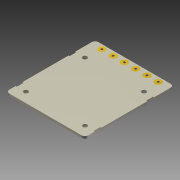
# Autodesk Inventor part: SLIPRING_SRG-1-6G_
Saved by Autodesk Inventor 2011 (Build 150239000, 239)
## iProperties
Created: 2012-05-23
Part Number: SLIPRING_SRG-1-6G_
Document SubType Name: Modeling
Designer: arihon
Density: 1 g/cm^3
Author: arihon
Autodesk Inventor part; units mm, degrees
ref_plane "YZ Plane" through (0, 0, 0) normal (1, 0, 0) x (0, 1, 0)
ref_plane "XZ Plane" through (0, 0, 0) normal (0, 1, 0) x (-1, 0, 0)
ref_plane "XY Plane" through (0, 0, 0) normal (0, 0, 1) x (1, 0, 0)
sketch "スケッチ1" plane through (0, 0, 0) normal (0, 0, 1) x (1, 0, 0)
  circle A0 centre (13.0815, -13.0815) radius 1
  circle A1 centre (-13.0815, 13.0815) radius 1
  circle A2 centre (13.0815, 13.0815) radius 1
  line L0 (-17.5, -17.5) -> (17.5, -17.5)
  line L1 (17.5, -17.5) -> (17.5, -13.2)
  line L2 (17.5, 22) -> (-17.5, 22)
  line L3 (-17.5, 22) -> (-17.5, 13.2505)
  line L4 (-17.0382, 13.2505) -> (-17.5, 13.2505)
  line L5 (-17.5, 13.2505) -> (-17.5, 13.2)
  line L6 (-17.5, 10.2) -> (-17.0382, 10.2)
  line L7 (-17.0382, 10.2) -> (-17.0382, 13.2505)
  line L8 (-17, -10.2) -> (-17.5, -10.2)
  line L9 (-17.5, -10.2) -> (-17.5, -13.2)
  line L10 (-17.5, -13.2) -> (-17, -13.2)
  line L11 (-17, -13.2) -> (-17, -10.2)
  line L12 (17.5, -10.2) -> (17, -10.2)
  line L13 (17, -10.2) -> (17, -13.2)
  line L14 (17, -13.2) -> (17.5, -13.2)
  line L15 (17.5, -13.2) -> (17.5, -10.2)
  line L16 (17.5, 13.2) -> (17, 13.2)
  line L17 (17, 13.2) -> (17, 10.2)
  line L18 (17, 10.2) -> (17.5, 10.2)
  line L19 (17.5, 10.2) -> (17.5, 13.2)
  line L20 (17, 13.2) -> (17.5, 13.2)
  line L21 (17.5, 13.2) -> (17.5, 22)
  line L22 (17.5, 10.2) -> (17.5, 13.2)
  line L23 (17.5, -10.2) -> (17.5, 10.2)
  line L24 (17.5, -13.2) -> (17.5, -10.2)
  line L25 (-17.5, -13.2) -> (-17.5, -17.5)
  line L26 (-17.5, -10.2) -> (-17.5, -13.2)
  line L27 (-17.5, 13.2505) -> (-17.5, 13.2)
  line L28 (-17.5, 13.2) -> (-17.5, 10.2)
  line L29 (-17.5, 10.2) -> (-17.5, -10.2)
  line L30 (-17.5, 13.2) -> (-17.5, 10.2)
  circle A3 centre (-13.0815, 13.0815) radius 1
  circle A4 centre (13.0815, 13.0815) radius 1
  circle A5 centre (-13.0815, -13.0815) radius 1
  circle A6 centre (13.0815, -13.0815) radius 1
  circle A7 centre (-13.0815, -13.0815) radius 1
  point P0 (0, 0)
  point P1 (0, 0)
  dimension "d0" = 39.5
  dimension "d1" = 2
  constraints: 63 end point, 40 parallel, 10 perpendicular, 8 centre point, 5 horizontal, 4 coincident, 3 concentric, 2 point on line
  measures "d0" distance of L2.end L0.start
  measures "d1" diameter of A5
extrude "押し出し1" add sketch "スケッチ1" along normal blind 1 contours L25 L10 L11 L8 L29 L6 L7 L4 L3 L2 L21 L16 L17 L18 L23 L12 L13 L14 L1 L0
fillet "フィレット1" radius 1.5 4 edges at (-17.5, -17.5, 0.5) (-17.5, 22, 0.5) (17.5, 22, 0.5) (17.5, -17.5, 0.5)
sketch "スケッチ2" plane through (0, 0, 1) normal (0, 0, 1) x (1, 0, 0)
  line L0 (17.5, 20.5) -> (17.5, 13.2) projected
  line L1 (-16, 22) -> (16, 22) projected
  line L2 (-17.5, 13.2505) -> (-17.5, 20.5) projected
  line L3 (16, -17.5) -> (-16, -17.5) projected
  line L4 (17.5, 20) -> (-17.5, 20)
  line L5 (0, 22) -> (0, -17.5)
  point P0 (0, 0)
  point P1 (2.5, 20)
  point P2 (7.5, 20)
  point P3 (12.5, 20)
  point P4 (-2.5, 20)
  point P5 (-7.5, 20)
  point P6 (-12.5, 20)
  dimension "d5" = 2
  dimension "d6" = 12.5
  dimension "d9" = 5
  dimension "d10" = 5
  constraints: 5 point on line, 4 end point, 3 symmetric about line, 2 midpoint, 1 parallel
  measures "d5" distance between parallel lines of L4 L1
  measures "d6" distance from line of point (12.5, 20) L5
  measures "d9" distance of point (12.5, 20) point (7.5, 20)
  measures "d10" distance of point (7.5, 20) point (2.5, 20)
hole "Hole1" at (2.5, 20, 1) at (7.5, 20, 1) at (12.5, 20, 1) at (-12.5, 20, 1) at (-7.5, 20, 1) at (-2.5, 20, 1) direction (0, 0, -1) diameter 1 end through all
sketch "スケッチ3" plane through (0, 0, 1) normal (0, 0, 1) x (1, 0, 0)
  circle A0 centre (-2.5, 20) radius 0.5 projected
  circle A1 centre (-7.5, 20) radius 0.5 projected
  circle A2 centre (-12.5, 20) radius 0.5 projected
  circle A3 centre (12.5, 20) radius 0.5 projected
  circle A4 centre (7.5, 20) radius 0.5 projected
  circle A5 centre (2.5, 20) radius 0.5 projected
  circle A6 centre (12.5, 20) radius 1.5
  circle A7 centre (7.5, 20) radius 1.5
  circle A8 centre (2.5, 20) radius 1.5
  circle A9 centre (-2.5, 20) radius 1.5
  circle A10 centre (-7.5, 20) radius 1.5
  circle A11 centre (-12.5, 20) radius 1.5
  point P0 (0, 0)
  dimension "d18" = 3
  dimension "d19" = 3
  dimension "d20" = 3
  dimension "d21" = 3
  dimension "d22" = 3
  dimension "d23" = 3
  constraints: 6 centre point, 6 coincident
  measures "d18" diameter of A6
  measures "d19" diameter of A7
  measures "d20" diameter of A8
  measures "d21" diameter of A9
  measures "d22" diameter of A10
  measures "d23" diameter of A11
extrude "押し出し2" add sketch "スケッチ3" along normal blind 0.01
equation "\"d10\" = d9"
equation "\"d19\" = d18"
equation "\"d20\" = d18"
equation "\"d21\" = d18"
equation "\"d22\" = d18"
equation "\"d23\" = d18"
